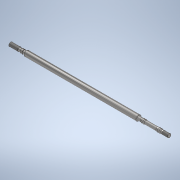
# Autodesk Inventor part: Шток_CPY
Saved by Autodesk Inventor 2021 (Build 250183000, 183)
## iProperties
Created: 2020-11-22
Part Number: Шток_CPY
Material: Сталь, углеродистая
Document SubType Name: Modeling
Designer: Тимоха
Mass: 25235.9 g
Surface Area: 2325.72 cm^2
Volume: 3214.77 cm^3
Density: 7.85 g/cm^3
Appearance: С умеренной полировкой
Author: Тимоха
Autodesk Inventor part; units mm, degrees
ref_plane "YZ Plane" through (0, 0, 0) normal (1, 0, 0) x (0, 1, 0)
ref_plane "XZ Plane" through (0, 0, 0) normal (0, 1, 0) x (-1, 0, 0)
ref_plane "XY Plane" through (0, 0, 0) normal (0, 0, 1) x (1, 0, 0)
sketch "Эскиз1" plane through (0, 0, 0) normal (0, 0, 1) x (1, 0, 0)
  line L0 (0, 0) -> (345, 0)
  line L1 (345, 0) -> (345, 20)
  line L2 (345, 20) -> (280, 20)
  line L3 (0, 0) -> (0, 22.5)
  line L4 (0, 22.5) -> (50, 22.5)
  line L5 (50, 22.5) -> (70, 22.5)
  line L6 (250, 22.5) -> (230, 22.5)
  line L7 (250, 22.5) -> (265, 18.9255)
  line L8 (265, 18.9255) -> (280, 20)
  line L9 (82.7171, 19.4628) -> (70, 22.5)
  line L10 (50, 22.5) -> (36.6597, 19.4628)
  line L11 (36.6597, 19.4628) -> (0, 19.4628)
  line L12 (230, 22.5) -> (211.3782, 19.4628)
  line L13 (211.3782, 19.4628) -> (82.7171, 19.4628)
  dimension "d0" = 345
  dimension "d1" = 20
  dimension "d2" = 65
  dimension "d5" = 22.5
  dimension "d6" = 50
  dimension "d7" = 20
  dimension "d8" = 20
  dimension "d15" = 30
  constraints: 28 end point, 3 horizontal, 3 perpendicular, 2 point on line, 1 vertical
  measures "d0" distance of L0.start L0.end
  measures "d1" distance of L0.end L1.end
  measures "d2" distance of L1.end L2.end
  measures "d5" distance of L0.start L3.end
  measures "d6" distance of L3.end L4.end
  measures "d7" distance of L4.end L5.end
  measures "d8" distance of L6.start L6.end
  measures "d15" horizontal distance of L2.end L6.start
revolve "Вращение1" add sketch "Эскиз1" angle 360 about axis through (0, 0, 0) along (1, 0, 0) contours L3 L11 L10 L5 L9 L13 L12 L6 L7 L8 L2 L1 L0
thread "Резьба1" size "M40x3" class "6g" standard "ANSI Metric M Profile" full length
sketch "Эскиз2" plane through (0, 0, 0) normal (-1, 0, 0) x (0, 0, 1)
  circle A0 centre (0, 0) radius 30
  dimension "d12" = 60
  constraints: 1 centre point, 1 coincident
  measures "d12" diameter of A0
extrude "Выдавливание1" add sketch "Эскиз2" along normal blind 1248.008
sketch "Эскиз3" plane through (-1248.008, 0, 0) normal (-1, 0, 0) x (0, 0, 1)
  circle A0 centre (0, 0) radius 22.5
  dimension "d16" = 45
  constraints: 1 centre point, 1 coincident
  measures "d16" diameter of A0
extrude "Выдавливание2" add sketch "Эскиз3" along normal blind 180
sketch "Эскиз4" plane through (0, 0, 0) normal (0, 0, 1) x (1, 0, 0)
  line L0 (-1248.008, 30) -> (-1248.008, -30) projected
  line L1 (-1428.008, 22.5) -> (-1428.008, -22.5) projected
  line L2 (-1248.008, -22.5) -> (-1248.008, 22.5) projected
  line L3 (-1248.008, 0) -> (-1248.008, 20)
  line L4 (-1248.008, 22.5) -> (-1248.008, 20)
  line L5 (-1248.008, 0) -> (-1248.008, -20.008)
  line L6 (-1248.008, -20.008) -> (-1278.008, -20.008)
  line L7 (-1278.008, -20.008) -> (-1280.5, -22.5)
  line L8 (-1280.5, -22.5) -> (-1300.5, -22.5)
  line L9 (-1248.008, -22.5) -> (-1428.008, -22.5) projected
  line L10 (-1300.5, -22.5) -> (-1302.992, -20.008)
  line L11 (-1331.0081, 27.5) -> (-1331.0081, -27.5) projected
  line L12 (-1302.992, -20.008) -> (-1328.5, -20.008)
  line L13 (-1328.5, -20.008) -> (-1331.0081, -22.5)
  line L14 (-1248.008, -22.5) -> (-1428.008, -22.5) projected
  line L15 (-1383, 0) -> (-1400.8637, 0)
  point P0 (-1280.5, -22.5)
  point P1 (-1248.008, -20.008)
  point P2 (-1348.9963, -21.5037)
  dimension "d31" = 30
  dimension "d32" = 135
  dimension "d33" = 20
  dimension "d34" = 135
  constraints: 20 end point, 5 point on line, 2 horizontal, 1 collinear, 1 midpoint, 1 perpendicular
  measures "d31" distance of L5.end L6.end
  measures "d32" angle of L7 L6
  measures "d33" distance of L7.end L8.end
  measures "d34" angle of L8 L10
revolve "Вращение2" cut sketch "Эскиз4" angle 360 about axis through (-1383, 0, 0) along (-1, 0, 0)
chamfer "Фаска1" distance 2 angle 45 1 edges at (-1428.008, 0, -22.5)
thread "Резьба2" size "M45x4.5" class "6g" standard "ANSI Metric M Profile" full length
chamfer "Фаска2" distance 2 angle 45 1 edges at (345, -20, 0)
fillet "Сопряжение2" radius 2 3 edges at (-1278.008, 20.008, 0) (-1302.992, 20.008, 0) (-1328.5, 20.008, 0)
